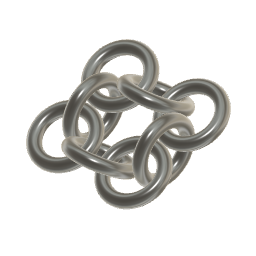
Chain Link (Autodesk Fusion 360 design; units mm, degrees)
Autodesk Fusion 360 part; units mm, degrees
torus "TorusPrimitive1" add centre line diameter 161.245 section diameter 40 placed x (1, 0, 0) y (0, 1, 0) z (0, 0, 1) at (0, 0, 0) makes body 1
delete_body "RemoveBody1" bodies 1
torus "TorusPrimitive2" add centre line diameter 110 section diameter 15 placed x (1, 0, 0) y (0, 1, 0) z (0, 0, 1) at (0, 0, 0) separate body makes body 2
sketch "Sketch5" plane through (0, 0, 0) normal (0, 0, 1) x (1, 0, 0)
move_body "MoveFace1" bodies 2 to x (0.906308, 0, -0.422618) y (0, 1, 0) z (0.422618, 0, 0.906308) at (0, 0, 0) on bodies 2
delete_face "DeleteFace1" 1 faces at (-49.0683, 32.3539, 20.0506) on bodies 2
torus "TorusPrimitive3" add centre line diameter 100 section diameter 10 placed x (1, 0, 0) y (0, 1, 0) z (0, 0, 1) at (0, 0, 0) separate body makes body 3
move_body "MoveFace2" bodies 3 to x (1, 0, 0) y (0, 0.939693, -0.34202) z (0, 0.34202, 0.939693) at (0, 0, 0) on bodies 3
torus "TorusPrimitive4" add centre line diameter 100 section diameter 10 placed x (0, 1, 0) y (0, 0, 1) z (1, 0, 0) at (0, 69.6571, -2.1466) separate body makes body 4
move_body "MoveFace3" bodies 4 to x (0.5, 0, 0.866025) y (0, 1, 0) z (-0.866025, 0, 0.5) at (-7.5636, -11.4886, -3.0892) on bodies 4
move_body "MoveFace4" bodies 3 to x (0.939693, 0.116978, 0.321394) y (-0.116978, 0.992945, -0.019382) z (-0.321394, -0.019382, 0.946747) at (0, 0, 0) on bodies 3
move_body "MoveFace5" bodies 4 to x (0.939693, 0, -0.34202) y (0, 1, 0) z (0.34202, 0, 0.939693) at (1.0796, 0, -2.2021) on bodies 4
copy_body "CopyPasteBodies1" bodies 4 3 makes body 5 makes body 6
move_body "Move1" bodies 5 6 to x (1, 0, 0) y (0, 1, 0) z (0, 0, 1) at (0, 125, 0)
delete_face "DeleteFace2" 1 faces at (-51.7292, -10.9349, -14.1196) on bodies 3
delete_face "DeleteFace3" 1 faces at (26.8308, 72.9831, -45.5971) on bodies 4
delete_face "DeleteFace4" 1 faces at (-5.8063, 174.6556, -22.2588) on bodies 6
delete_face "DeleteFace5" 1 faces at (-40.3433, 200.5893, 34.4578) on bodies 5
torus "TorusPrimitive5" add centre line diameter 25 section diameter 6 placed x (1, 0, 0) y (0, 1, 0) z (0, 0, 1) at (0, 0, 0) separate body makes body 7
copy_body "CopyPasteBodies2" bodies 7 makes body 8
move_body "Move2" bodies 8 to x (1, 0, 0) y (0, 1, 0) z (0, 0, 1) at (6, 0, 0)
copy_body "CopyPasteBodies3" bodies 8 7 makes body 9 makes body 10
move_body "Move3" bodies 9 10 to x (1, 0, 0) y (0, 1, 0) z (0, 0, 1) at (13, 0, 0)
move_body "MoveFace6" bodies 7 to x (1, 0, 0) y (0, 0.939693, 0.34202) z (0, -0.34202, 0.939693) at (0, 0, 0) on bodies 7
move_body "MoveFace7" bodies 8 to x (1, 0, 0) y (0, 0.939693, -0.34202) z (0, 0.34202, 0.939693) at (0, 0, 0) on bodies 8
delete_face "DeleteFace6" 1 faces at (28.3, -0.7636, 1.0261) on bodies 10
delete_face "DeleteFace7" 1 faces at (34.3, -0.7636, 1.0261) on bodies 9
copy_body "CopyPasteBodies4" bodies 7 8 makes body 11 makes body 12
move_body "Move4" bodies 11 12 to x (1, 0, 0) y (0, 1, 0) z (0, 0, 1) at (13, 0, 0)
copy_body "CopyPasteBodies5" bodies 11 12 makes body 13 makes body 14
move_body "Move5" bodies 13 14 to x (1, 0, 0) y (0, 1, 0) z (0, 0, 1) at (13, 0, 0)
delete_face "DeleteFace8" 4 faces at (27.3952, -5.2744, -0.8278) (34.3, -0.3666, 1.2253) (34.9424, -12.039, -3.2899) (17.1546, -3.2012, 2.2571) on bodies 11 12 13 14
move_body "MoveFace8" bodies 7 to x (1, 0, 0) y (0, 1, 0) z (0, 0, 1) at (-2, 0, 0) on bodies 7
move_body "MoveFace9" bodies 7 to x (1, 0, 0) y (0, 1, 0) z (0, 0, 1) at (-5, 0, 0) on bodies 7
move_body "MoveFace10" bodies 8 to x (1, 0, 0) y (0, 0.984808, -0.173648) z (0, 0.173648, 0.984808) at (0, 0, 0) on bodies 8
move_body "MoveFace11" bodies 7 to x (1, 0, 0) y (0, 0.984808, 0.173648) z (0, -0.173648, 0.984808) at (0, 0, 0) on bodies 7
copy_body "CopyPasteBodies6" bodies 7 8 makes body 15 makes body 16
move_body "Move6" bodies 15 16 to x (1, 0, 0) y (0, 1, 0) z (0, 0, 1) at (27, 0, 0)
delete_face "DeleteFace9" 1 faces at (35.3, -1.1743, 0.5068) on bodies 15
delete_face "DeleteFace10" 1 faces at (18.6048, 5.0505, -1.7311) on bodies 16
move_body "Move7" bodies 7 to x (1, 0, 0) y (0, 1, 0) z (0, 0, 1) at (-1, 0, 0)
copy_body "CopyPasteBodies7" bodies 7 8 makes body 17 makes body 18
move_body "Move8" bodies 17 18 to x (1, 0, 0) y (0, 1, 0) z (0, 0, 1) at (28, 0, 0)
copy_body "CopyPasteBodies8" bodies 17 18 makes body 19 makes body 20
move_body "Move9" bodies 19 20 to x (1, 0, 0) y (0, 1, 0) z (0, 0, 1) at (28, 0, 0)
copy_body "CopyPasteBodies9" bodies 19 makes body 21
move_body "Move10" bodies 21 to x (1, 0, 0) y (0, 1, 0) z (0, 0, 1) at (27, -1.7321, -1)
delete_face "DeleteFace11" 1 faces at (89.1162, -6.3723, -4.8638) on bodies 21
copy_body "CopyPasteBodies10" bodies 19 makes body 22
move_body "Move11" bodies 22 to x (1, 0, 0) y (0, 1, 0) z (0, 0, 1) at (28, 0, 0)
move_body "Move12" bodies 22 19 17 7 to x (1, 0, 0) y (0, 1, 0) z (0, 0, 1) at (0, -1.1684, -0.8727)
copy_body "CopyPasteBodies11" bodies 20 makes body 23
move_body "Move13" bodies 23 to x (0, 0.5, 0.866025) y (-0.5, 0.75, -0.433013) z (-0.866025, -0.433013, 0.25) at (62, -31, -53.6936)
move_body "Move14" bodies 23 to x (1, 0, 0) y (0, 1, 0) z (0, 0, 1) at (12.8543, 17.3485, -1.8181)
delete_face "DeleteFace12" 1 faces at (63.3, -2.3427, -0.3659) on bodies 19
delete_face "DeleteFace13" 1 faces at (76.1162, -5.6663, 2.0866) on bodies 20
delete_face "DeleteFace14" 1 faces at (90.1162, -5.8086, -4.7365) on bodies 22
move_body "Move15" bodies 23 to x (1, 0, 0) y (0, 1, 0) z (0, 0, 1) at (-39, 0, 0)
move_body "Move16" bodies 18 17 23 to x (1, 0, 0) y (0, 1, 0) z (0, 0, 1) at (4, 0, 0)
move_body "Move17" bodies 18 23 to x (1, 0, 0) y (0, 1, 0) z (0, 0, 1) at (4, 0, 0)
move_body "MoveFace12" bodies 23 to x (1, 0, 0) y (0, 1, 0) z (0, 0, 1) at (-19, 0, 0) on bodies 23
move_body "Move18" bodies 23 to x (1, 0, 0) y (0, 1, 0) z (0, 0, 1) at (-1, 0, 0)
move_body "MoveFace13" bodies 23 to x (1, 0, 0) y (0, 1, 0) z (0, 0, 1) at (0.1682, -2.1102, 1.381) on bodies 23
move_body "Move19" bodies 23 to x (1, 0, 0) y (0, 1, 0) z (0, 0, 1) at (-0.0432, -0.9838, 2.2747)
move_body "Move20" bodies 18 to x (1, 0, 0) y (0, 1, 0) z (0, 0, 1) at (0.4786, 0.1023, 0.0141)
move_body "Move21" bodies 8 7 to x (1, 0, 0) y (0, 1, 0) z (0, 0, 1) at (-0.5, 0, 0)
delete_face "DeleteFace15" 1 faces at (-22.8952, -6.2189, -2.6038) on bodies 7
copy_body "CopyPasteBodies12" bodies 17 23 makes body 24 makes body 25
move_body "Move22" bodies 24 25 to x (1, 0, 0) y (0, 1, 0) z (0, 0, 1) at (37, 0, 0)
copy_body "CopyPasteBodies13" bodies 8 17 18 24 makes body 26 makes body 27 makes body 28 makes body 29
move_body "Move23" bodies 26 27 28 29 to x (1, 0, 0) y (0, 1, 0) z (0, 0, 1) at (-0.0047, 28.5414, 10.7135)
move_body "MoveFace14" bodies 24 to x (1, 0, 0) y (0, 1, 0) z (0, 0, 1) at (-1.3528, 0.8737, -0.584) on bodies 24
move_body "MoveFace15" bodies 27 to x (1, 0, 0) y (0, 1, 0) z (0, 0, 1) at (-0.129, 1.0097, 0.6862) on bodies 27
move_body "MoveFace16" bodies 29 to x (1, 0, 0) y (0, 1, 0) z (0, 0, 1) at (0, 1.7321, 1) on bodies 29
move_body "MoveFace17" bodies 17 to x (1, 0, 0) y (0, 1, 0) z (0, 0, 1) at (0.2954, 0.0664, -1.3622) on bodies 17
move_body "MoveFace18" bodies 8 18 to x (1, 0, 0) y (0, 1, 0) z (0, 0, 1) at (0.3426, -1.7774, -3.3044) on bodies 8 18
move_body "MoveFace19" bodies 8 18 to x (1, 0, 0) y (0, 1, 0) z (0, 0, 1) at (0.1248, 0.4911, 0.6485) on bodies 8 18
delete_face "DeleteFace16" 1 faces at (8.1555, 41.0935, 2.2817) on bodies 26
delete_face "DeleteFace17" 1 faces at (1.0885, 11.8026, -9.028) on bodies 8
equation "d12 = inner_diam"
equation "d13 = outer_diam"
equation "inner_diam = 6 mm"
equation "outer_diam = 25 mm"
